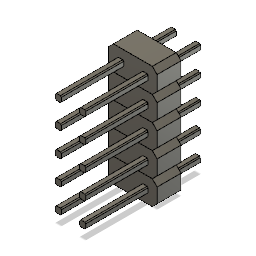
Electrical unit v1 (Autodesk Fusion 360 design; units mm, degrees)
Autodesk Fusion 360 part; units mm, degrees
sketch "Sketch1" plane through (0, 0, 0) normal (0, 0, 1) x (1, 0, 0)
  line L0 (0.325, -0.325) -> (-0.325, -0.325)
  line L1 (-0.325, -0.325) -> (-0.325, 0.325)
  line L2 (-0.325, 0.325) -> (0.325, 0.325)
  line L3 (0.325, 0.325) -> (0.325, -0.325)
  line L4 (0.325, -0.325) -> (-0.325, 0.325) construction
  line L5 (-0.325, -0.325) -> (0.325, 0.325) construction
  dimension "d2" = 0.65
  dimension "d3" = 0.65
  constraint horizontal L0
  constraint perpendicular L0 L1
  constraint parallel L0 L2
  constraint parallel L1 L3
  constraint coincident L4 origin
  constraint coincident L5 origin
  measures "d2" distance of L0.start L0.end
  measures "d3" distance of L0.end L1.end
extrude "Extrude1" add sketch "Sketch1" along normal blind 12 makes body 1
chamfer "Chamfer1" distance 0.1 angle 45 1 edges at (0.325, -0.325, 6) on bodies 1
chamfer "Chamfer2" distance 0.1 angle 45 3 edges at (-0.325, -0.325, 6) (-0.325, 0.325, 6) (0.325, 0.325, 6) on bodies 1
pattern_linear "R-Pattern1" count 2 spacing 2.54 along (1, 0, 0) of bodies 1 makes body 2
sketch "Sketch2" plane through (0, 0, 0) normal (0, 0, -1) x (-1, 0, 0)
  line L0 (-0.225, 0.325) -> (-0.325, 0.225)
  line L1 (-0.325, 0.225) -> (-0.325, -0.225)
  line L2 (-0.325, -0.225) -> (-0.225, -0.325)
  line L3 (-0.225, -0.325) -> (0.225, -0.325)
  line L4 (0.225, -0.325) -> (0.325, -0.225)
  line L5 (0.325, -0.225) -> (0.325, 0.225)
  line L6 (0.325, 0.225) -> (0.225, 0.325)
  line L7 (0.225, 0.325) -> (-0.225, 0.325)
  line L8 (-0.225, -0.325, 0) -> (-0.225, -0.325, -3) construction
  line L9 (0, 0) -> (-1.27, 0) construction
  line L10 (-3.81, -1.27, -3) -> (1.27, -1.27, -3)
  line L11 (1.27, -1.27, -3) -> (1.27, 1.27, -3)
  line L12 (1.27, 1.27, -3) -> (-3.81, 1.27, -3)
  line L13 (-3.81, 1.27, -3) -> (-3.81, -1.27, -3)
  point P0 (-1.27, 0)
  point P1 (-1.27, 0)
  dimension "d14" = 1.27
  constraint coincident L2.end L3.start
  constraint coincident L9.start origin
  constraint parallel L3 L9
  constraint coincident P1 P0
  measures "d14" distance of L9.start P1
extrude "Extrude2" add sketch "Sketch2" against normal blind 2.5 contours L10 L11 L12 L13 in plane through (0, 0, 3) normal (0, 0, -1) bodies 1 2
chamfer "Chamfer3" distance 0.5 angle 45 4 edges at (3.81, 1.27, 4.25) (-1.27, 1.27, 4.25) (3.81, -1.27, 4.25) (-1.27, -1.27, 4.25) on bodies 1
pattern_linear "R-Pattern2" count 1 spacing 0 along (1, 0, 0) count 5 spacing 2.54 along (0, 1, 0) of bodies 1 makes body 3 at (0.9217, 1.585, 5.5) makes body 4 at (1.6183, 4.125, 5.5) makes body 5 at (1.6183, 6.665, 5.5) makes body 6 at (0.9217, 9.205, 5.5)
